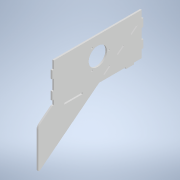
# Autodesk Inventor part: Soporte_Rodamientos
Saved by Autodesk Inventor 2020.1 (Build 241239000, 239)
## iProperties
Created: 2019-12-08
Part Number: Soporte_Rodamientos
Material: Generic
Document SubType Name: Modeling
Designer: Daniel
Density: 1 g/cm^3
Appearance: Default
Author: Daniel
Autodesk Inventor part; units mm, degrees
ref_plane "YZ Plane" through (0, 0, 0) normal (1, 0, 0) x (0, 1, 0)
ref_plane "XZ Plane" through (0, 0, 0) normal (0, 1, 0) x (-1, 0, 0)
ref_plane "XY Plane" through (0, 0, 0) normal (0, 0, 1) x (1, 0, 0)
sketch "Sketch1" plane through (0, 0, 0) normal (1, 0, 0) x (0, 1, 0)
  line L0 (-40, 84) -> (40, 84)
  line L1 (40, 84) -> (40, -84)
  line L2 (40, -84) -> (-40, -84)
  line L3 (-40, -84) -> (-40, 84)
  line L4 (-40, 84) -> (40, -84) construction
  line L5 (40, 84) -> (-40, -84) construction
  circle A0 centre (5, 0) radius 17.5
  point P0 (0, 0)
  dimension "d0" = 35
  dimension "d5" = 35
  dimension "d6" = 80
  dimension "d7" = 168
  dimension "d8" = 84
  constraints: 12 end point, 2 midpoint, 2 parallel, 1 centre point, 1 horizontal, 1 perpendicular
  measures "d0" diameter of A0
  measures "d5" distance from line of L1 A0.centre
  measures "d6" distance of L1.end L2.end
  measures "d7" distance of L0.end L1.end
  measures "d8" distance from line of L0 A0.centre
extrude "Extrusion1" add sketch "Sketch1" along normal blind 3
sketch "Sketch2" plane through (3, 0, 0) normal (1, 0, 0) x (0, 0, -1)
  circle A0 centre (0, 5) radius 17.5 projected
  circle A1 centre (0, 5) radius 21.5 construction
  line L0 (0, -66.71) -> (0, 54.4228) construction
  line L1 (0, 5) -> (51.042, 5) construction
  point P0 (0, 0)
  point P1 (21.5, 5)
  point P2 (-10.75, 23.6195)
  point P3 (-10.75, -13.6195)
  dimension "d11" = 43
  dimension "d14" = 360
  constraints: 4 end point, 2 vertical, 1 coincident, 1 horizontal, 1 horizontal alignment, 1 point on line, 9 other
hole "Hole1" at (3, 5, -21.5) at (3, 23.6195, 10.75) at (3, -13.6195, 10.75) direction (-1, 0, 0) diameter 3 depth 10 tip angle 118
sketch "Sketch5" plane through (3, 0, 0) normal (1, 0, 0) x (0, 0, -1)
  circle A0 centre (0, 5) radius 17.5 projected
  circle A1 centre (0, 5) radius 31 construction
  line L0 (-114, -127.2132) -> (84, 27.4814)
  line L1 (84, -40) -> (84, 40) projected
  line L2 (-84, -40) -> (84, -40) projected
  line L3 (-112.153, -129.5772) -> (84, 23.6743)
  line L4 (76.1199, 17.5177) -> (74.2729, 19.8817)
  line L5 (64.2997, 8.2828) -> (62.4527, 10.6468)
  line L6 (-84, 40) -> (-84, -40) projected
  line L7 (-114, -55.0733) -> (-87, -33.9786)
  line L8 (-112.153, -129.5772) -> (-114, -127.2132)
  line L9 (-114, -127.2132) -> (-114, -55.0733)
  line L10 (84, 40) -> (-84, 40) projected
  line L11 (38.2954, -12.034) -> (36.4484, -9.67)
  line L12 (50.1155, -2.7991) -> (48.2686, -0.4351)
  line L13 (12.291, -32.3509) -> (10.444, -29.9868)
  line L14 (24.1112, -23.116) -> (22.2642, -20.7519)
  line L15 (-84, -33.9786) -> (-87, -33.9786)
  line L16 (-87, -33.9786) -> (-87, 40) construction
  line L17 (-84, 40) -> (-87, 40) construction
  point P0 (0, 0)
  point P1 (11.0887, -29.6815)
  point P2 (12.9357, -32.0456)
  point P3 (2.5006, -40)
  dimension "d24" = 62
  dimension "d25" = 38
  dimension "d27" = 3
  dimension "d28" = 10
  dimension "d33" = 30
  dimension "d37" = 15
  dimension "d40" = 3
  dimension "d43" = 33
  dimension "d54" = 3
  dimension "d56" = 55
  constraints: 28 end point, 7 point on line, 3 perpendicular, 2 horizontal, 2 parallel, 1 centre point, 1 coincident, 1 vertical, 13 other
  measures "d24" diameter of A1
  measures "d25" angle of L2 L0
  measures "d27" distance between parallel lines of L0 L3
  measures "d28" distance from line of L3.end L4
  measures "d33" distance from line of L6 L0.start
  measures "d37" distance between parallel lines of L4 L5
  measures "d40" distance edge to line of A1 L0
  measures "d43" distance of L5.start L11.start
  measures "d54" distance between parallel lines of L6 L16
  measures "d56" distance from line of L0 L15.start
extrude "Extrusion2" cut sketch "Sketch5" against normal blind 10 contours L0 L14 L3 L13 | L0 L12 L3 L11 | L0 L4 L3 L5
extrude "Extrusion3" add sketch "Sketch5" against normal up to surface (3 mm away) contours L2 L3 L8 L0 | L0 L9 L7 L15 L6 L2
fillet "Fillet1" radius 10 1 edges at (1.5, -55.0733, 114)
sketch "Sketch7" plane through (3, 0, 0) normal (1, 0, 0) x (0, 0, -1)
  line L0 (-84, 40) -> (-84, -33.9786) projected
  line L1 (2.5006, -40) -> (84, -40) projected
  line L2 (-29, -40) -> (-64, -40)
  line L3 (-64, -40) -> (-64, -43)
  line L4 (-64, -43) -> (-29, -43)
  line L5 (-29, -43) -> (-29, -40)
  point P0 (0, 0)
  dimension "d49" = 3
  dimension "d50" = 35
  dimension "d51" = 20
  constraints: 8 end point, 2 parallel, 1 horizontal, 1 perpendicular, 1 point on line
  measures "d49" distance of L2.end L3.end
  measures "d50" distance of L3.end L4.end
  measures "d51" distance between parallel lines of L3 L0
extrude "Extrusion4" cut sketch "Sketch7" against normal blind 10
sketch "Sketch8" plane through (3, 0, 0) normal (1, 0, 0) x (0, 0, -1)
  line L0 (84, -25) -> (87, -25)
  line L1 (87, -25) -> (87, -10)
  line L2 (87, -10) -> (84, -10)
  line L3 (84, -10) -> (84, -25)
  line L4 (84, -40) -> (84, 40) projected
  line L5 (84, -40) -> (84, 40) projected
  line L6 (84, 0) -> (0, 0) construction
  line L7 (84, 25) -> (87, 25)
  line L8 (87, 25) -> (87, 10)
  line L9 (87, 10) -> (84, 10)
  line L10 (84, 10) -> (84, 25)
  line L11 (84, 40) -> (-84, 40) construction
  line L12 (0, 40) -> (0, 0) construction
  line L13 (-84, -25) -> (-87, -25)
  line L14 (-87, -25) -> (-87, -10)
  line L15 (-87, -10) -> (-84, -10)
  line L16 (-84, -10) -> (-84, -25)
  line L17 (-87, 25) -> (-87, 10)
  line L18 (-87, 10) -> (-84, 10)
  line L19 (-84, 25) -> (-87, 25)
  line L20 (-84, 10) -> (-84, 25)
  line L21 (69, -40) -> (54, -40)
  line L22 (54, -40) -> (54, -43)
  line L23 (54, -43) -> (69, -43)
  line L24 (69, -43) -> (69, -40)
  line L25 (2.5006, -40) -> (84, -40) projected
  point P0 (-84, 0)
  dimension "d0" = 35
  dimension "d57" = 3
  dimension "d58" = 15
  dimension "d59" = 15
  dimension "d62" = 3
  dimension "d63" = 15
  dimension "d64" = 15
  constraints: 44 end point, 13 symmetric about line, 4 parallel, 3 horizontal, 3 perpendicular, 2 collinear, 2 midpoint
  measures "d57" distance of L0.start L0.end
  measures "d58" distance of L0.end L1.end
  measures "d59" distance from line of L0 L4.start
  measures "d62" distance of L21.end L22.end
  measures "d63" distance of L22.end L23.end
  measures "d64" distance between parallel lines of L4 L24
extrude "Extrusion5" add sketch "Sketch8" against normal up to surface (3 mm away)
equation "\"d8\" = 0.5 * d7"
body "Solid1"
